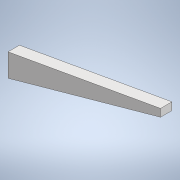
# Autodesk Inventor part: Leg
Saved by Autodesk Inventor 2022 (Build 260153000, 153)
## iProperties
Created: 2022-01-06
Part Number: Leg
Material: Generic
Document SubType Name: Modeling
Designer: dangl
Density: 1 g/cm^3
Appearance: Default
Author: dangl
Autodesk Inventor part; units mm, degrees
ref_plane "YZ Plane" through (0, 0, 0) normal (1, 0, 0) x (0, 1, 0)
ref_plane "XZ Plane" through (0, 0, 0) normal (0, 1, 0) x (-1, 0, 0)
ref_plane "XY Plane" through (0, 0, 0) normal (0, 0, 1) x (1, 0, 0)
sketch "Sketch1" plane through (0, 0, 0) normal (0, 0, 1) x (1, 0, 0)
  line L0 (12.7, -443.8005) -> (12.7, -36.275) projected
  line L1 (12.7, -101.6) -> (520.7, -10.875)
  line L2 (520.7, -10.875) -> (520.7, -36.275)
  line L3 (520.7, -36.275) -> (12.7, -177.8)
  line L4 (12.7, -177.8) -> (12.7, -101.6)
  point P0 (0, 0)
  dimension "d0" = 508
  dimension "d1" = 25.4
  dimension "d2" = 76.2
  dimension "d3" = 101.6
  constraints: 8 end point, 2 point on line, 1 vertical
  measures "d0" distance between parallel lines of L2 L0
  measures "d1" distance of L1.end L2.end
  measures "d2" distance of L1.start L3.end
  measures "d3" vertical distance of point (0, 0) L1.start
extrude "Extrusion1" add sketch "Sketch1" along normal mid plane 38.1
body "Solid1"
